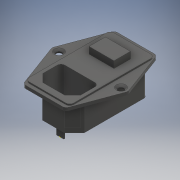
# Autodesk Inventor part: Plug+prise
Saved by Autodesk Inventor 2017 (Build 210142000, 142)
## iProperties
Part Number: Plug+prise
Material: Plastique ABS
Document SubType Name: Modeling
Designer: Adrien MARY
Density: 1.06 g/cm^3
Appearance: Lisse - Blanc(1)
Mass: 22.7371 g
Surface Area: 94.0762 cm^2
Volume: 21.4501 cm^3
Stock Number: 1410-03-06
Project: 1410 LaserShow
Author: Adrien MARY
Autodesk Inventor part; units mm, degrees
ref_plane "YZ Plane" through (0, 0, 0) normal (1, 0, 0) x (0, 1, 0)
ref_plane "XZ Plane" through (0, 0, 0) normal (0, 1, 0) x (-1, 0, 0)
ref_plane "XY Plane" through (0, 0, 0) normal (0, 0, 1) x (1, 0, 0)
sketch "Esquisse1" plane through (0, 0, 0) normal (0, 0, 1) x (1, 0, 0)
  line L0 (-13.4, -23.5) -> (13.4, -23.5)
  line L1 (13.4, -23.5) -> (13.4, 23.5)
  line L2 (13.4, 23.5) -> (-13.4, 23.5)
  line L3 (-13.4, 23.5) -> (-13.4, -23.5)
  line L4 (-13.4, -23.5) -> (13.4, 23.5) construction
  line L5 (13.4, -23.5) -> (-13.4, 23.5) construction
  point P0 (0, 0)
  dimension "d0" = 26.8
  dimension "d1" = 47
  constraints: 12 end point, 2 midpoint, 2 parallel, 1 horizontal, 1 perpendicular
  measures "d0" distance of L2.end L1.end
  measures "d1" distance of L1.end L0.end
extrude "Extrusion1" add sketch "Esquisse1" along normal blind 18
chamfer "Chanfrein1" distance 6.5 angle 45 2 edges at (-13.4, -23.5, 9) (13.4, -23.5, 9)
sketch "Esquisse2" plane through (0, 0, 18) normal (0, 0, 1) x (1, 0, 0)
  line L0 (-24.4, 0) -> (-13.5, 29.4)
  line L1 (-13.5, 29.4) -> (13.5, 29.4)
  line L2 (13.5, 29.4) -> (24.4, 0)
  line L3 (24.4, 0) -> (13.5, -29.4)
  line L4 (13.5, -29.4) -> (-13.5, -29.4)
  line L5 (-13.5, -29.4) -> (-24.4, 0)
  point P0 (0, 0)
  point P1 (0, 29.4)
  point P2 (0, -29.4)
  dimension "d7" = 58.8
  dimension "d8" = 29.4
  dimension "d9" = 48.8
  dimension "d10" = 24.4
  dimension "d11" = 27
  dimension "d12" = 27
  constraints: 12 end point, 2 equal length, 2 midpoint, 2 vertical alignment, 1 horizontal, 1 parallel
  measures "d7" distance between parallel lines of L4 L1
  measures "d8" distance from line of point (0, 0) L1
  measures "d9" distance of L2.end L0.start
  measures "d10" distance of point (0, 0) L2.end
  measures "d11" distance of L0.end L1.end
  measures "d12" distance of L3.end L4.end
extrude "Extrusion2" add sketch "Esquisse2" along normal blind 1.9
sketch "Esquisse3" plane through (0, 0, 19.9) normal (0, 0, 1) x (1, 0, 0)
  line L0 (-14.25, -27.25) -> (14.25, -27.25)
  line L1 (14.25, -27.25) -> (14.25, 27.25)
  line L2 (14.25, 27.25) -> (-14.25, 27.25)
  line L3 (-14.25, 27.25) -> (-14.25, -27.25)
  point P0 (0, 0)
  point P1 (-14.25, 0)
  point P2 (0, 27.25)
  dimension "d15" = 28.5
  dimension "d16" = 54.5
  constraints: 8 end point, 2 midpoint, 2 parallel, 1 horizontal, 1 horizontal alignment, 1 perpendicular, 1 vertical alignment
  measures "d15" distance of L1.end L2.end
  measures "d16" distance of L0.end L1.end
extrude "Extrusion3" add sketch "Esquisse3" along normal blind 0.9
sketch "Esquisse4" plane through (0, 0, 20.8) normal (0, 0, 1) x (1, 0, 0)
  line L0 (-7.1, -23.25) -> (7.1, -23.25)
  line L1 (12.1, -18.25) -> (12.1, -9)
  line L2 (9.6, -6.5) -> (-9.6, -6.5)
  line L3 (-12.1, -9) -> (-12.1, -18.25)
  line L4 (-14.25, -27.25) -> (14.25, -27.25) projected
  line L5 (-7.1, -23.25) -> (-12.1, -18.25)
  line L6 (7.1, -23.25) -> (12.1, -18.25)
  arc A0 (-9.6, -6.5) -> (-12.1, -9) centre (-9.6, -9) ccw
  arc A1 (12.1, -9) -> (9.6, -6.5) centre (9.6, -9) ccw
  point P0 (0, 0)
  point P1 (-12.1, -23.25)
  point P2 (12.1, -23.25)
  point P3 (-12.1, -6.5)
  point P4 (0, -6.5)
  dimension "d19" = 24.2
  dimension "d20" = 16.75
  dimension "d21" = 4
  dimension "d22" = 5
  dimension "d23" = 5
  dimension "d24" = 5
  dimension "d25" = 5
  dimension "d26" = 2.5
  constraints: 12 end point, 6 point on line, 4 point on circle, 4 tangent, 2 centre point, 2 parallel, 1 equal radius, 1 horizontal, 1 midpoint, 1 perpendicular, 1 vertical alignment
  measures "d19" distance between parallel lines of L1 L3
  measures "d20" distance of point (-12.1, -6.5) point (-12.1, -23.25)
  measures "d21" distance between parallel lines of L4 L0
  measures "d22" distance of L0.start point (-12.1, -23.25)
  measures "d23" distance of L3.end point (-12.1, -23.25)
  measures "d24" distance of L0.end point (12.1, -23.25)
  measures "d25" distance of L1.start point (12.1, -23.25)
  measures "d26" radius of A0
extrude "Extrusion4" cut sketch "Esquisse4" against normal blind 18.11
sketch "Esquisse5" plane through (0, 0, 20.8) normal (0, 0, 1) x (1, 0, 0)
  line L0 (-8, 7.4) -> (8, 7.4)
  line L1 (8, 7.4) -> (8, 17.9)
  line L2 (8, 17.9) -> (-8, 17.9)
  line L3 (-8, 17.9) -> (-8, 7.4)
  line L4 (14.25, 27.25) -> (-14.25, 27.25) projected
  point P0 (0, 0)
  point P1 (0, 7.4)
  dimension "d29" = 16
  dimension "d30" = 10.5
  dimension "d31" = 9.35
  constraints: 8 end point, 2 parallel, 1 horizontal, 1 midpoint, 1 perpendicular, 1 vertical alignment
  measures "d29" distance of L1.end L2.end
  measures "d30" distance of L0.end L1.end
  measures "d31" distance between parallel lines of L4 L2
extrude "Extrusion5" add sketch "Esquisse5" along normal blind 4.3
sketch "Esquisse6" plane through (0, 0, 0) normal (0, 0, -1) x (-1, 0, 0)
  line L0 (-2.35, -19.2) -> (2.35, -19.2)
  line L1 (2.35, -19.2) -> (2.35, -18.5)
  line L2 (2.35, -18.5) -> (-2.35, -18.5)
  line L3 (-2.35, -18.5) -> (-2.35, -19.2)
  line L4 (4.7, -9.5) -> (9.4, -9.5)
  line L5 (9.4, -9.5) -> (9.4, -8.8)
  line L6 (9.4, -8.8) -> (4.7, -8.8)
  line L7 (4.7, -8.8) -> (4.7, -9.5)
  line L8 (4.7, 3.2) -> (9.4, 3.2)
  line L9 (9.4, 3.2) -> (9.4, 3.9)
  line L10 (9.4, 3.9) -> (4.7, 3.9)
  line L11 (4.7, 3.9) -> (4.7, 3.2)
  line L12 (6.9, -23.5) -> (-6.9, -23.5) projected
  line L13 (13.4, 23.5) -> (13.4, -17) projected
  point P0 (0, 0)
  point P1 (0, -19.2)
  dimension "d34" = 4.7
  dimension "d35" = 0.7
  dimension "d38" = 0.7
  dimension "d40" = 0.7
  dimension "d41" = 4.3
  dimension "d42" = 14
  dimension "d43" = 12
  dimension "d44" = 4
  dimension "d45" = 4.7
  constraints: 24 end point, 6 parallel, 3 horizontal, 3 perpendicular, 2 point on line, 1 midpoint, 1 vertical alignment
  measures "d34" distance of L0.start L0.end
  measures "d35" distance between parallel lines of L2 L0
  measures "d38" distance between parallel lines of L10 L8
  measures "d40" distance between parallel lines of L6 L4
  measures "d41" distance between parallel lines of L12 L0
  measures "d42" distance between parallel lines of L12 L4
  measures "d43" distance between parallel lines of L8 L6
  measures "d44" distance between parallel lines of L13 L5
  measures "d45" distance of L5.end L6.end
extrude "Extrusion6" add sketch "Esquisse6" along normal blind 8
sketch "Esquisse7" plane through (0, 0, 0) normal (0, 0, -1) x (-1, 0, 0)
  line L0 (-6.525, 17.2) -> (-1.825, 17.2)
  line L1 (-1.825, 17.2) -> (-1.825, 18)
  line L2 (-1.825, 18) -> (-6.525, 18)
  line L3 (-6.525, 18) -> (-6.525, 17.2)
  line L4 (-6.525, 8.9) -> (-1.825, 8.9)
  line L5 (-1.825, 8.9) -> (-1.825, 9.7)
  line L6 (-1.825, 9.7) -> (-6.525, 9.7)
  line L7 (-6.525, 9.7) -> (-6.525, 8.9)
  line L8 (1.825, 16.5) -> (6.525, 16.5)
  line L9 (6.525, 16.5) -> (6.525, 15.7)
  line L10 (6.525, 15.7) -> (1.825, 15.7)
  line L11 (1.825, 15.7) -> (1.825, 16.5)
  line L12 (1.825, 9.9) -> (6.525, 9.9)
  line L13 (6.525, 9.9) -> (6.525, 10.7)
  line L14 (6.525, 10.7) -> (1.825, 10.7)
  line L15 (1.825, 10.7) -> (1.825, 9.9)
  line L16 (-13.4, 23.5) -> (13.4, 23.5) projected
  point P0 (0, 0)
  dimension "d48" = 4.7
  dimension "d49" = 4.7
  dimension "d50" = 0.8
  dimension "d51" = 0.8
  dimension "d52" = 0.8
  dimension "d53" = 0.8
  dimension "d54" = 7.5
  dimension "d55" = 5
  dimension "d56" = 3.65
  dimension "d57" = 1.825
  dimension "d58" = 5.5
  dimension "d60" = 1.5
  constraints: 32 end point, 8 parallel, 4 horizontal, 4 perpendicular, 4 point on line
  measures "d48" distance of L1.end L2.end
  measures "d49" distance of L13.end L14.end
  measures "d50" distance between parallel lines of L2 L0
  measures "d51" distance between parallel lines of L6 L4
  measures "d52" distance between parallel lines of L14 L12
  measures "d53" distance between parallel lines of L8 L10
  measures "d54" distance between parallel lines of L0 L6
  measures "d55" distance between parallel lines of L14 L10
  measures "d56" distance between parallel lines of L5 L15
  measures "d57" distance from line of point (0, 0) L5
  measures "d58" distance between parallel lines of L16 L2
  measures "d60" distance between parallel lines of L8 L2
extrude "Extrusion7" add sketch "Esquisse7" along normal blind 4
sketch "Esquisse8" plane through (0, 0, 19.9) normal (0, 0, 1) x (1, 0, 0)
  point P0 (0, 0)
  point P1 (-19.905, 0)
  point P2 (19.905, 0)
  dimension "d63" = 39.81
  dimension "d64" = 19.905
  constraints: 2 horizontal alignment
  measures "d63" distance of point (19.905, 0) point (-19.905, 0)
  measures "d64" distance of point (0, 0) point (-19.905, 0)
hole "Perçage1" at (-19.905, 0, 19.9) at (19.905, 0, 19.9) direction (0, 0, -1) diameter 3.6 end through all countersink diameter 6 countersink angle 90
fillet "Congé1" radius 2.5 12 edges at (-13.5, 29.4, 18.95) (-13.5, -29.4, 18.95) (13.5, -29.4, 18.95) (13.5, 29.4, 18.95) (24.4, 0, 18.95) (-24.4, 0, 18.95) (-14.25, 27.25, 20.35) (14.25, 27.25, 20.35) (-14.25, -27.25, 20.35) (14.25, -27.25, 20.35) (13.4, 23.5, 9) (-13.4, 23.5, 9)
equation "\"d8\" = 0.5 * d7"
equation "\"d10\" = 0.5 * d9"
equation "\"d12\" = d11"
equation "\"d23\" = d22"
equation "\"d24\" = d22"
equation "\"d25\" = d24"
equation "\"d38\" = d35"
equation "\"d40\" = d35"
equation "\"d45\" = d34"
equation "\"d49\" = d48"
equation "\"d51\" = d50"
equation "\"d52\" = d51"
equation "\"d53\" = d52"
equation "\"d57\" = 0.5 * d56"
equation "\"d64\" = 0.5 * d63"
equation "\"pi\" = 3.141593"
equation "\"nombredor\" = 1.61803"
